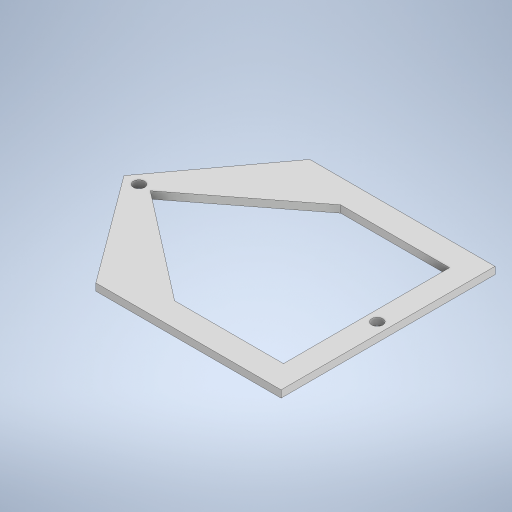
# Autodesk Inventor part: CO-1-02-fuseMount
Saved by Autodesk Inventor 2024 (Build 280153000, 153)
## iProperties
Created: 2023-03-23
Part Number: CO-1-02-fuseMount
Material: Generic
Document SubType Name: Modeling
Designer: beh5452
Density: 1 g/cm^3
Appearance: Default
Author: beh5452
Autodesk Inventor part; units mm, degrees
ref_plane "YZ Plane" through (0, 0, 0) normal (1, 0, 0) x (0, 1, 0)
ref_plane "XY Plane" through (0, 0, 0) normal (0, 0, 1) x (1, 0, 0)
ref_plane "Work Plane4" through (0, 32, 0) normal (0, 1, 0) x (-1, 0, 0)
sketch "Sketch1" plane through (0, 0, 0) normal (0, 1, 0) x (-1, 0, 0)
  line L0 (33.75, 44.75) -> (-33.75, 44.75)
  line L1 (-33.75, 44.75) -> (-33.75, -44.75)
  line L2 (-33.75, -44.75) -> (33.75, -44.75)
  line L3 (33.75, -44.75) -> (33.75, 44.75)
  line L4 (21.75, -36.75) -> (-21.75, -36.75)
  line L5 (21.75, 36.75) -> (-21.75, 36.75)
  line L6 (21.75, 36.75) -> (21.75, -36.75)
  line L7 (-21.75, 36.75) -> (-21.75, -36.75)
  line L8 (33.75, -41.75) -> (-33.75, -41.75)
  line L9 (33.75, 41.75) -> (-33.75, 41.75)
  line L10 (-6.7955, 36.75) -> (21.75, 0)
  line L11 (21.75, 0) -> (0, -36.75)
  point P0 (0, 0)
  point P1 (-33.75, 0)
  dimension "d0" = 83.5
  dimension "d1" = 3
  dimension "d2" = 3
  dimension "d4" = 5
  dimension "d5" = 5
  dimension "d6" = 12
  dimension "d7" = 12
  dimension "d8" = 67.5
  dimension "d9" = 33.75
  dimension "d10" = 41.75
  constraints: 24 end point, 7 perpendicular, 5 point on line, 3 horizontal, 3 midpoint
  measures "d0" distance between parallel lines of L8 L9
  measures "d1" distance between parallel lines of L0 L9
  measures "d2" distance between parallel lines of L8 L2
  measures "d4" distance between parallel lines of L9 L5
  measures "d5" distance between parallel lines of L8 L4
  measures "d6" distance between parallel lines of L3 L6
  measures "d7" distance between parallel lines of L7 L1
  measures "d8" distance from line of point (-33.75, 0) L3
  measures "d9" distance from line of point (0, 0) L1
  measures "d10" distance from line of point (0, 0) L8
sketch "Sketch2" plane through (0, 32, 0) normal (0, 1, 0) x (1, 0, 0)
  line L0 (33.75, -44.75) -> (33.75, -41.75)
  line L1 (33.75, -41.75) -> (-33.75, -41.75)
  line L2 (-33.75, -41.75) -> (-33.75, -44.75)
  line L3 (-33.75, -44.75) -> (33.75, -44.75)
  line L4 (-33.75, 44.75) -> (-33.75, 41.75)
  line L5 (-33.75, 41.75) -> (33.75, 41.75)
  line L6 (33.75, 41.75) -> (33.75, 44.75)
  line L7 (33.75, 44.75) -> (-33.75, 44.75)
  line L8 (33.75, -41.75) -> (33.75, 41.75) projected
  line L9 (-33.75, 34.75) -> (24.75, 34.75)
  line L10 (-33.75, -34.75) -> (24.75, -34.75)
  line L11 (24.75, -34.75) -> (24.75, 0)
  line L12 (24.75, 0) -> (24.75, 34.75)
  line L13 (-33.75, -34.75) -> (-65.75, 0)
  line L14 (-65.75, 0) -> (-33.75, 34.75)
  line L15 (33.75, 44.75) -> (33.75, 0)
  line L16 (33.75, -41.75) -> (33.75, -44.75) projected
  line L17 (33.75, 0) -> (33.75, -44.75)
  line L18 (-33.75, -44.75) -> (-76.75, 0)
  line L19 (-33.75, 44.75) -> (-33.75, 41.75) projected
  line L20 (-76.75, 0) -> (-33.75, 44.75)
  line L21 (-33.75, -44.75) -> (-43.75, -44.75)
  line L22 (-43.75, -44.75) -> (-76.75, 0)
  line L23 (-33.75, 44.75) -> (-43.75, 44.75)
  line L24 (-43.75, 44.75) -> (-76.75, 0)
  line L25 (-20.8207, 34.75) -> (-65.75, 0)
  line L26 (-65.75, 0) -> (-20.8207, -34.75)
  line L27 (-33.75, -44.75) -> (33.75, -44.75)
  line L28 (-33.75, 44.75) -> (33.75, 44.75)
  point P0 (0, 0)
  dimension "d18" = 7
  dimension "d19" = 7
  dimension "d20" = 110.5
  dimension "d21" = 90.5
  dimension "d42" = 9
  dimension "d78" = 10
  dimension "d79" = 10
  dimension "d88" = 9.639
  dimension "d89" = 9.639
  constraints: 40 end point, 4 horizontal alignment, 3 equal length, 2 collinear, 2 horizontal, 2 point on line, 1 perpendicular
  measures "d18" distance between parallel lines of L5 L9
  measures "d19" distance between parallel lines of L1 L10
  measures "d20" distance of L15.end L18.end
  measures "d21" distance of L13.end L11.end
  measures "d42" distance between parallel lines of L11 L17
  measures "d78" distance of L2.end L21.end
  measures "d79" distance of L4.start L23.end
  measures "d88" angle of L26 L13
  measures "d89" angle of L14 L25
extrude "Extrusion3" add sketch "Sketch2" along normal blind 3 contours L3 L2 L1 L0 | L1 L2 L18 L20 L4 L5 L8 | L21 L22 L18 | L24 L23 L20 | L5 L4 L7 L6 | L9 L25 L14 | L26 L10 L13
sketch "Sketch3" plane through (0, 32, 0) normal (0, 1, 0) x (1, 0, 0)
  circle A0 centre (29.25, 0) radius 4.5
  circle A1 centre (-70.45, 0) radius 4.5
  circle A2 centre (-70.45, 0) radius 2.35
  circle A3 centre (29.25, 0) radius 2.35
  line L0 (33.75, -44.75) -> (33.75, 44.75)
  point P0 (0, 0)
  dimension "d24" = 9
  dimension "d27" = 4.7
  dimension "d43" = 99.7
  dimension "d44" = 4.5
  constraints: 4 centre point, 2 coincident, 2 end point, 2 equal radius, 2 horizontal alignment
  measures "d24" diameter of A1
  measures "d27" diameter of A2
  measures "d43" distance of A1.centre A0.centre
  measures "d44" distance from line of L0 A0.centre
extrude "Extrusion5" cut sketch "Sketch3" along normal blind 3 contours A2 | A3
equation "\"d9\" = 0.5 * d8"
equation "\"d10\" = 0.5 * d0"
equation "\"d19\" = d18"
equation "\"d44\" = 0.5 * d24"
equation "\"d2\" = d1"
equation "\"d5\" = d4"
equation "\"d7\" = d6"
body "Solid1"
